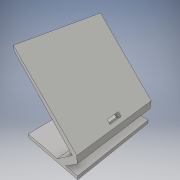
# Autodesk Inventor part: proto_1b
Saved by Autodesk Inventor 2016 (Build 200138000, 138)
## iProperties
Created: 2017-07-19
Part Number: proto_1b
Material: Generic
Document SubType Name: Modeling
Designer: Logan
Density: 1 g/cm^3
Appearance: Default
Author: Logan
Autodesk Inventor part; units mm, degrees
ref_plane "YZ Plane" through (0, 0, 0) normal (1, 0, 0) x (0, 1, 0)
ref_plane "XZ Plane" through (0, 0, 0) normal (0, 1, 0) x (-1, 0, 0)
ref_plane "XY Plane" through (0, 0, 0) normal (0, 0, 1) x (1, 0, 0)
sketch "Sketch1" plane through (0, 0, 0) normal (0, 0, 1) x (1, 0, 0)
  line L0 (-44.9013, 44.9013) -> (44.9013, -44.9013)
  line L1 (-44.9013, 44.9013) -> (82.0987, 44.9013) construction
  line L2 (-44.9013, 44.9013) -> (-44.9013, 38.5513)
  line L3 (44.9013, -44.9013) -> (44.9013, -57.6013)
  line L4 (44.9013, -57.6013) -> (-44.9013, 38.5513)
  line L5 (44.9013, -57.6013) -> (44.9013, -76.6513) construction
  line L6 (-44.9013, 38.5513) -> (-44.9013, -76.6513) construction
  line L7 (-44.9013, 38.5513) -> (70.3013, 38.5513) construction
  line L8 (-44.9013, -76.6513) -> (44.9013, -76.6513)
  line L9 (-44.9013, -76.6513) -> (-44.9013, -83.0013)
  line L10 (44.9013, -76.6513) -> (44.9013, -83.0013)
  line L11 (44.9013, -76.6513) -> (51.2513, -76.6513) construction
  line L12 (-44.9013, -83.0013) -> (44.9013, -83.0013)
  line L13 (44.9013, -57.6013) -> (25.8513, -76.6513)
  line L14 (44.9013, -57.6013) -> (71.842, -57.6013) construction
  line L15 (44.9013, -57.6013) -> (37.9664, -50.1761) construction
  line L16 (37.9664, -50.1761) -> (11.4912, -76.6513)
  line L17 (37.9664, -50.1761) -> (75.408, -50.1761) construction
  point P0 (0, 0)
  point P1 (0, 0)
  dimension "d0" = 127
  dimension "d1" = 45
  dimension "d2" = 6.35
  dimension "d4" = 19.05
  dimension "d5" = 12.7
  dimension "d6" = 90
  dimension "d7" = 6.35
  dimension "d8" = 90
  dimension "d9" = 135
  dimension "d10" = 10.16
  dimension "d11" = 135
  constraints: 36 end point, 6 equal length, 6 horizontal, 4 point on line, 2 perpendicular, 1 coincident, 1 midpoint, 1 vertical
  measures "d0" distance of L0.start L0.end
  measures "d1" angle of L0 L1
  measures "d2" distance of L0.start L2.end
  measures "d4" distance of L3.end L5.end
  measures "d5" distance of L0.end L3.end
  measures "d6" angle of L6 L7
  measures "d7" distance of L6.end L9.end
  measures "d8" angle of L10 L11
  measures "d9" angle of L13 L14
  measures "d10" distance of L3.end L15.end
  measures "d11" angle of L16 L17
extrude "Extrusion1" add sketch "Sketch1" against normal blind 127
sketch "Sketch4" plane through (37.9664, -50.1761, -127) normal (-0.7308, -0.6826, 0) x (0, 0, 1)
  line L0 (0, -1.2778) -> (0, 0) projected
  line L1 (127, 0) -> (127, -1.2778) projected
  line L2 (0, 0) -> (127, 0) construction
  line L3 (127, 0) -> (0, 0) projected
  line L4 (63.5, 0) -> (63.5, 5.08) construction
  line L5 (63.5, 0) -> (68.58, 0) construction
  line L6 (53.975, 11.43) -> (73.025, 11.43)
  line L7 (73.025, 11.43) -> (73.025, 5.08)
  line L8 (73.025, 5.08) -> (53.975, 5.08)
  line L9 (53.975, 5.08) -> (53.975, 11.43)
  point P0 (127, 62.5845)
  dimension "d22" = 5.08
  dimension "d23" = 90
  dimension "d24" = 19.05
  dimension "d25" = 6.35
  constraints: 14 end point, 3 horizontal, 3 perpendicular, 2 midpoint, 2 parallel
  measures "d22" distance of L4.end L4.start
  measures "d23" angle of L5 L4
  measures "d24" distance of L7.end L8.end
  measures "d25" distance of L6.end L7.end
extrude "Extrusion4" cut sketch "Sketch4" against normal up to next
body "Solid1"
